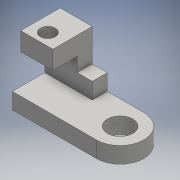
# Autodesk Inventor part: 240503_3Dsketch07
Saved by Autodesk Inventor 2016 (Build 200138000, 138)
## iProperties
Created: 2024-05-03
Part Number: 240503_3Dsketch07
Material: 일반
Document SubType Name: Modeling
Designer: pc
Density: 1 g/cm^3
Appearance: 기본값
Author: pc
Autodesk Inventor part; units mm, degrees
ref_plane "YZ Plane" through (0, 0, 0) normal (1, 0, 0) x (0, 1, 0)
ref_plane "XZ Plane" through (0, 0, 0) normal (0, 1, 0) x (-1, 0, 0)
ref_plane "XY Plane" through (0, 0, 0) normal (0, 0, 1) x (1, 0, 0)
sketch "스케치1" plane through (0, 0, 0) normal (0, 0, 1) x (1, 0, 0)
  line L0 (25.8992, -14.5721) -> (-25.8992, -14.5721)
  line L1 (-25.8992, -14.5721) -> (-25.8992, 14.5721)
  line L2 (-25.8992, 14.5721) -> (25.8992, 14.5721)
  line L3 (25.8992, -14.5721) -> (-25.8992, 14.5721) construction
  line L4 (-25.8992, -14.5721) -> (25.8992, 14.5721) construction
  arc A0 (25.8992, -14.5721) -> (25.8992, 14.5721) centre (25.8992, 0) ccw
  circle A1 centre (25.8992, 0) radius 7.8142
  point P0 (0, 0)
  constraints: 10 end point, 2 centre point, 2 midpoint, 2 point on circle, 1 coincident, 1 horizontal, 1 parallel, 1 perpendicular, 1 tangent
extrude "돌출1" add sketch "스케치1" along normal blind 10
sketch "스케치2" plane through (0, 0, 10) normal (0, 0, 1) x (1, 0, 0)
  line L0 (-25.8992, 14.5721) -> (-25.8992, -14.5721) projected
  line L1 (-25.8992, 14.5721) -> (3.3382, 14.5721)
  line L2 (3.3382, 14.5721) -> (3.3382, 5.3954)
  line L3 (3.3382, 5.3954) -> (-25.8992, 5.3954)
  line L4 (-25.8992, 5.3954) -> (-25.8992, 14.5721)
  point P0 (0, 0)
  constraints: 8 end point, 2 parallel, 1 horizontal, 1 perpendicular
extrude "돌출2" add sketch "스케치2" along normal blind 10
sketch "스케치3" plane through (0, 0, 20) normal (0, 0, 1) x (1, 0, 0)
  line L0 (-25.8992, 5.3954) -> (3.3382, 5.3954) projected
  line L1 (-25.7105, 14.6501) -> (-5.9667, 14.6501)
  line L2 (-5.9667, 14.6501) -> (-5.9667, 5.3954)
  line L3 (-5.9667, 5.3954) -> (-25.7105, 5.3954)
  line L4 (-25.7105, 5.3954) -> (-25.7105, 14.6501)
  point P0 (0, 0)
  constraints: 8 end point, 2 parallel, 1 horizontal, 1 perpendicular, 1 point on line
extrude "돌출3" add sketch "스케치3" along normal blind 20
sketch "스케치4" plane through (-25.8992, 5.3954, 10) normal (0, -1, 0) x (1, 0, 0)
  line L0 (0.1887, 30) -> (19.9325, 30) projected
  line L1 (19.9325, 10) -> (19.9325, 30) projected
  line L2 (0.1887, 30) -> (19.9325, 30)
  line L3 (19.9325, 30) -> (19.9325, 18.6928)
  line L4 (19.9325, 18.6928) -> (0.1887, 18.6928)
  line L5 (0.1887, 18.6928) -> (0.1887, 30)
  point P0 (25.8992, -10)
  constraints: 8 end point, 2 parallel, 1 horizontal, 1 perpendicular, 1 point on line
extrude "돌출4" add sketch "스케치4" along normal blind 15
sketch "스케치5" plane through (0, 0, 40) normal (0, 0, 1) x (1, 0, 0)
  circle A0 centre (-16.4269, -2.2401) radius 4.6425
  point P0 (0, 0)
  constraints: 1 centre point
extrude "돌출5" cut sketch "스케치5" against normal blind 15
